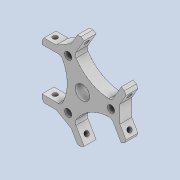
# Autodesk Inventor part: wheel_2_ori
Saved by Autodesk Inventor 2020 (Build 240168000, 168)
## iProperties
Created: 2022-01-11
Part Number: wheel_2_ori
Material: Generic
Document SubType Name: Modeling
Designer: Shuang Peng
Density: 1 g/cm^3
Appearance: Default
Author: Shuang Peng
Autodesk Inventor part; units mm, degrees
ref_plane "YZ Plane" through (0, 0, 0) normal (1, 0, 0) x (0, 1, 0)
ref_plane "XZ Plane" through (0, 0, 0) normal (0, 1, 0) x (-1, 0, 0)
ref_plane "XY Plane" through (0, 0, 0) normal (0, 0, 1) x (1, 0, 0)
sketch "Sketch1" plane through (0, 0, 0) normal (0, 0, 1) x (1, 0, 0)
  circle A0 centre (-3, -5.1962) radius 0.75 projected
  circle A1 centre (-3, 5.1962) radius 0.75 projected
  circle A2 centre (6, 0) radius 0.75 projected
  circle A3 centre (0, 0) radius 1.5 projected
  arc A4 (0, -6.5) -> (5.6292, -3.25) centre (0, 0) ccw projected
  arc A5 (-1.299, -4.25) -> (0, -6.5) centre (0, -5) ccw projected
  line L0 (-1.299, -4.25) -> (-0.5701, -2.9875) projected
  arc A6 (0.2114, -2.491) -> (-0.5701, -2.9875) centre (0.2959, -3.4875) ccw projected
  arc A7 (0.2114, -2.491) -> (2.0516, -1.4286) centre (0, 0) ccw projected
  arc A8 (2.8723, -1) -> (2.0516, -1.4286) centre (2.8723, -2) ccw projected
  line L1 (2.8723, -1) -> (4.3301, -1) projected
  arc A9 (5.6292, -3.25) -> (4.3301, -1) centre (4.3301, -2.5) ccw projected
  arc A10 (-5.6292, 3.25) -> (-5.6292, -3.25) centre (0, 0) ccw projected
  arc A11 (-3.0311, 3.25) -> (-5.6292, 3.25) centre (-4.3301, 2.5) ccw projected
  line L2 (-3.0311, 3.25) -> (-2.3022, 1.9875) projected
  arc A12 (-2.263, 1.0625) -> (-2.3022, 1.9875) centre (-3.1682, 1.4875) ccw projected
  arc A13 (-2.263, 1.0625) -> (-2.263, -1.0625) centre (0, 0) ccw projected
  arc A14 (-2.3022, -1.9875) -> (-2.263, -1.0625) centre (-3.1682, -1.4875) ccw projected
  line L3 (-2.3022, -1.9875) -> (-3.0311, -3.25) projected
  arc A15 (-5.6292, -3.25) -> (-3.0311, -3.25) centre (-4.3301, -2.5) ccw projected
  arc A16 (5.6292, 3.25) -> (0, 6.5) centre (0, 0) ccw projected
  arc A17 (4.3301, 1) -> (5.6292, 3.25) centre (4.3301, 2.5) ccw projected
  line L4 (4.3301, 1) -> (2.8723, 1) projected
  arc A18 (2.0516, 1.4286) -> (2.8723, 1) centre (2.8723, 2) ccw projected
  arc A19 (2.0516, 1.4286) -> (0.2114, 2.491) centre (0, 0) ccw projected
  arc A20 (-0.5701, 2.9875) -> (0.2114, 2.491) centre (0.2959, 3.4875) ccw projected
  line L5 (-0.5701, 2.9875) -> (-1.299, 4.25) projected
  arc A21 (0, 6.5) -> (-1.299, 4.25) centre (0, 5) ccw projected
  circle A22 centre (0, 0) radius 7.2 projected
  circle A23 centre (0, 0) radius 10
  line L6 (-10, 0) -> (-7, 0)
  line L7 (0, 0) -> (-10, 0)
  line L8 (-7, 0) -> (-7, 7.1414)
  line L9 (-7, 0) -> (-7, -7.1414)
  line L10 (-7, 0) -> (-7, -0.3577)
  line L11 (-7, 0) -> (-7, -4.5)
  line L12 (-7, -4.5) -> (-8.9303, -4.5)
  line L13 (-7, 0) -> (-7, 4.5)
  line L14 (-7, 4.5) -> (-8.9303, 4.5)
  line L15 (-7, -4.5) -> (-7, -5.2)
  line L16 (-8.5, -5.9) -> (-8.5, -4.5)
  line L17 (-8.5, -4.5) -> (-5.5, -4.5)
  line L18 (-5.5, -4.5) -> (-5.5, -5.9)
  line L19 (-5.5, -5.9) -> (-8.5, -5.9)
  line L20 (-8.5, -5.9) -> (-5.5, -4.5) construction
  line L21 (-8.5, -4.5) -> (-5.5, -5.9) construction
  line L22 (-5.5, -4.5) -> (-4.5, -4.5)
  line L23 (-4.5, -4.5) -> (0, 0)
  line L24 (-7, 4.5) -> (-8.9303, 4.5)
  line L25 (-8.5, 5.9) -> (-8.5, 4.5)
  line L26 (-8.5, 4.5) -> (-5.5, 4.5)
  line L27 (-5.5, 4.5) -> (-5.5, 5.9)
  line L28 (-5.5, 5.9) -> (-8.5, 5.9)
  line L29 (-5.5, 4.5) -> (-4.5, 4.5)
  line L30 (-4.5, 4.5) -> (0, 0)
  line L31 (9.3595, -4.4112) -> (8.1471, -5.1112)
  line L32 (7.8595, -1.8131) -> (9.3595, -4.4112)
  line L33 (6.6471, -2.5131) -> (7.8595, -1.8131)
  line L34 (8.1471, -5.1112) -> (6.6471, -2.5131)
  line L35 (6.6471, -2.5131) -> (6.1471, -1.6471)
  line L36 (6.1471, -1.6471) -> (0, 0)
  line L37 (-1.6471, -6.1471) -> (0, 0)
  line L38 (0.3529, -9.6112) -> (-1.1471, -7.0131)
  line L39 (-1.1471, -7.0131) -> (-1.6471, -6.1471)
  line L40 (-1.1471, -7.0131) -> (-2.3595, -7.7131)
  line L41 (-2.3595, -7.7131) -> (-0.8595, -10.3112)
  line L42 (-0.8595, -10.3112) -> (0.3529, -9.6112)
  line L43 (-0.3971, -8.3122) -> (0.568, -9.9839)
  line L44 (-0.8595, 10.3112) -> (0.3529, 9.6112)
  line L45 (-2.3595, 7.7131) -> (-0.8595, 10.3112)
  line L46 (-1.1471, 7.0131) -> (-2.3595, 7.7131)
  line L47 (0.3529, 9.6112) -> (-1.1471, 7.0131)
  line L48 (-1.1471, 7.0131) -> (-1.6471, 6.1471)
  line L49 (-1.6471, 6.1471) -> (0, 0)
  line L50 (6.1471, 1.6471) -> (0, 0)
  line L51 (8.1471, 5.1112) -> (6.6471, 2.5131)
  line L52 (6.6471, 2.5131) -> (6.1471, 1.6471)
  line L53 (6.6471, 2.5131) -> (7.8595, 1.8131)
  line L54 (7.8595, 1.8131) -> (9.3595, 4.4112)
  line L55 (9.3595, 4.4112) -> (8.1471, 5.1112)
  line L56 (7.3971, 3.8122) -> (8.3623, 5.4839)
  line L57 (-2.3595, -7.7131) -> (-5.5, -5.9)
  line L58 (-5.5, 5.9) -> (-2.3595, 7.7131)
  line L59 (7.8595, -1.8131) -> (7.8595, 1.8131)
  arc A24 (-4.5, -4.5) -> (-4.5, 4.5) centre (-11.7111, 0) ccw
  arc A25 (6.1471, -1.6471) -> (-1.6471, -6.1471) centre (5.8556, -10.1421) ccw
  arc A26 (-1.6471, 6.1471) -> (6.1471, 1.6471) centre (5.8556, 10.1421) ccw
  point P0 (0, 0)
  point P1 (-8.5, -5.2678)
  point P2 (-8.074, -5.9)
  point P3 (-1.0725, -9.9423)
  point P4 (-0.3121, -9.9951)
  point P5 (8.8121, -4.7273)
  point P6 (9.1466, -4.0423)
  point P7 (9.1466, 4.0423)
  point P8 (8.8121, 4.7273)
  point P9 (-0.3121, 9.9951)
  point P10 (-1.0725, 9.9423)
  point P11 (-8.074, 5.9)
  point P12 (-8.5, 5.2678)
  dimension "d0" = 20
  dimension "d1" = 3
  dimension "d2" = 4.5
  dimension "d3" = 4.5
  dimension "d4" = 0.7
  dimension "d5" = 1.4
  dimension "d6" = 3
  dimension "d7" = 1
  dimension "d10" = 360
  dimension "d12" = 8.5
  dimension "d15" = 360
  constraints: 108 end point, 11 point on circle, 5 symmetric about line, 4 centre point, 4 perpendicular, 4 point on line, 3 horizontal, 3 parallel, 2 midpoint, 2 vertical, 1 coincident, 92 other
  measures "d0" diameter of A23
  measures "d1" distance of L6.start L6.end
  measures "d2" distance of L6.end L11.end
  measures "d3" distance of L6.end L13.end
  measures "d4" distance of L11.end L15.end
  measures "d5" distance of L16.start L16.end
  measures "d6" distance of L16.end L17.end
  measures "d7" distance of L17.end L22.end
  measures "d12" radius of A24
extrude "Extrusion1" add sketch "Sketch1" along normal blind 2 contours A3 L50 L4 A17 L52 L53 A22 L33 L35 L36 A9 L1 | A3 L49 L5 A20 A19 A18 L4 L50 | L36 L1 A8 A7 A6 L0 L37 A3 | A3 L30 L2 A11 L29 L27 A22 L46 L48 L49 A21 L5 | L50 A17 L4 | L4 A18 A19 A20 L5 L49 A21 A26 A17 L50 | L37 L0 A5 L39 L40 A22 L18 L22 L23 A15 L3 A3 | L36 A9 A25 A5 L37 L0 A6 A7 A8 L1 | L1 A9 L36 | A3 L7 A13 A12 L2 L30 | L5 A21 L49 | A17 A26 L50 | A3 L23 L3 A14 A13 L7 | L37 A5 L0 | L36 A25 A9 | L30 A11 L2 | L2 A12 A13 L7 A24 A11 L30 | L49 A26 A21 | A13 A14 L3 L23 A15 A24 L7 | L3 A15 L23 | A5 A25 L37 | A11 A24 L30 | L51 A22 L53 | L23 A24 A15 | L33 A22 L34 | L46 A22 L47 | L51 L55 A23 L54 L53 A22 | L53 L59 L33 A22 | L38 A22 L40 | L33 L32 A23 L31 L34 A22 | L26 A22 L27 | L46 L45 A23 L44 L47 A22 | A22 L27 L58 L46 | L18 A22 L17 | L38 L42 A23 L41 L40 A22 | L40 L57 L18 A22 | L26 L8 L28 L27 A22 | A22 L18 L19 L9 L17 | L14 L25 A23 L28 L8 | L9 L19 A23 L16 L12
sketch "Sketch2" plane through (-8.5, -4.5, 0) normal (0, 1, 0) x (1, 0, 0)
  line L0 (4, 0) -> (0, 0) projected
  line L1 (0, 0) -> (0, -2) projected
  line L2 (4, -2) -> (0, -2) projected
  line L3 (4, 0) -> (4, -2) projected
  line L4 (0, -1) -> (1.5, -1)
  circle A0 centre (1.5, -1) radius 0.5
  point P0 (8.5, 0)
  dimension "d19" = 1.5
  dimension "d20" = 1
  constraints: 2 end point, 1 centre point, 1 coincident, 1 horizontal, 1 midpoint
  measures "d19" distance of L4.start L4.end
  measures "d20" diameter of A0
extrude "Extrusion2" cut sketch "Sketch2" against normal mid plane 200 contours A0
pattern_circular "Circular Pattern1" count 3 over 360 about axis through (0, 0, 0) along (0, 0, 1) of "Extrusion2"
thicken "Thicken1" operation add thickness 0.25 both sides no extend neighbours yes toward (0, 0, 1) faces at (3.6699, -0.5977, 2)
thicken "Thicken2" operation add thickness 0.25 both sides no extend neighbours yes toward (0, 0, -1) faces at (3.6699, -0.5977, 0)
fillet "Fillet1" radius 1 6 edges at (-4.5, 4.5, 1) (-4.5, -4.5, 1) (-1.6471, -6.1471, 1) (6.1471, -1.6471, 1) (6.1471, 1.6471, 1) (-1.6471, 6.1471, 1)
body "Solid1"
